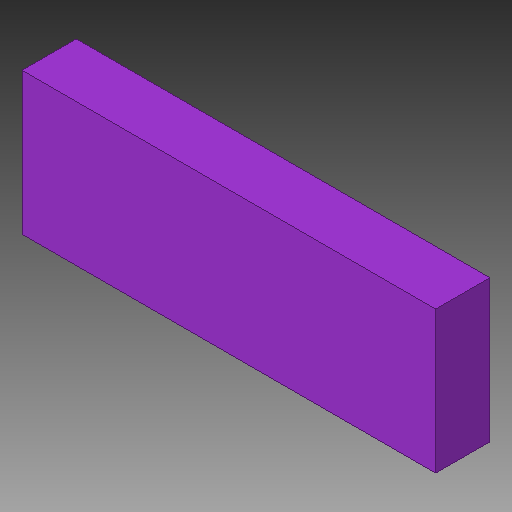
# Autodesk Inventor part: 1X03
Saved by Autodesk Inventor 2018 (Build 220112000, 112)
## iProperties
Created: 2015-11-24
Part Number: 1X03
Material: Generic
Document SubType Name: Modeling
Designer: PhillipD
Density: 1 g/cm^3
Appearance: 1X03, 1X03
Author: PhillipD
Autodesk Inventor part; units mm, degrees
ref_plane "YZ Plane" through (0, 0, 0) normal (1, 0, 0) x (0, 1, 0)
ref_plane "XZ Plane" through (0, 0, 0) normal (0, 1, 0) x (-1, 0, 0)
ref_plane "XY Plane" through (0, 0, 0) normal (0, 0, 1) x (1, 0, 0)
sketch "1X03, 1X03_53" plane through (0, 0, 0) normal (0, 0, 1) x (1, 0, 0)
  line L0 (-3.81, 1.3462) -> (3.81, 1.3462)
  line L1 (3.81, 1.3462) -> (3.81, -1.27)
  line L2 (3.81, -1.27) -> (-3.81, -1.27)
  line L3 (-3.81, -1.27) -> (-3.81, 1.3462)
  constraints: 8 end point
extrude "Extrusion1" add sketch "1X03, 1X03_53" along normal blind 1
body "Solid1"
